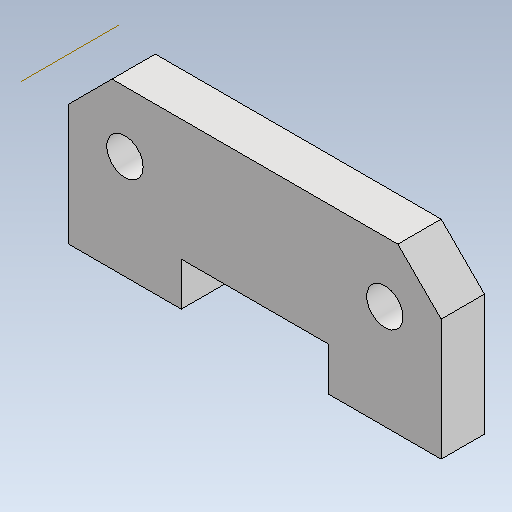
# Autodesk Inventor part: bed-hinge
Saved by Autodesk Inventor 2025 (Build 290162000, 162)
## iProperties
Created: 2025-08-20
Part Number: bed-hinge
Material: Generic
Document SubType Name: Modeling
Designer: HP
Density: 1 g/cm^3
Appearance: Default
Author: HP
Autodesk Inventor part; units mm, degrees
ref_plane "YZ Plane" through (0, 0, 0) normal (1, 0, 0) x (0, 1, 0)
ref_plane "XZ Plane" through (0, 0, 0) normal (0, 1, 0) x (-1, 0, 0)
ref_plane "XY Plane" through (0, 0, 0) normal (0, 0, 1) x (1, 0, 0)
sketch "Sketch1" plane through (0, 0, 0) normal (0, 0, 1) x (1, 0, 0)
  line L0 (6.5, 0) -> (-36.5, 0)
  line L1 (0, 14) -> (0, 0) construction
  circle A0 centre (0, 7) radius 2.1
  line L2 (-6.5, -5) -> (6.5, -5)
  line L3 (6.5, -5) -> (6.5, 14)
  line L4 (6.5, 0) -> (-6.5, 0)
  line L5 (-6.5, 0) -> (-6.5, -5)
  line L6 (-6.5, -5) -> (6.5, 0) construction
  line L7 (6.5, -5) -> (-6.5, 0) construction
  circle A1 centre (-30, 7) radius 2.1
  line L8 (-30, 14) -> (-30, 0) construction
  line L9 (6.5, 14) -> (-36.5, 14)
  line L10 (-36.5, -5) -> (-23.5, -5)
  line L11 (-23.5, -5) -> (-23.5, 0)
  line L12 (-23.5, 0) -> (-36.5, 0)
  line L13 (-36.5, 14) -> (-36.5, -5)
  line L14 (-36.5, -5) -> (-23.5, 0) construction
  line L15 (-23.5, -5) -> (-36.5, 0) construction
  line L16 (-15, 14) -> (-15, 0) construction
  point P0 (0, -2.5)
  point P1 (-6.5, 0)
  point P2 (-30, -2.5)
  point P3 (-23.5, 0)
  point P4 (-36.5, 0)
  point P5 (-30, 7)
  point P6 (-23.5, 0)
  point P7 (-6.5, 0)
  dimension "d1" = 4.2
  dimension "d4" = 7
  dimension "d5" = 5
  dimension "d6" = 13
  dimension "d8" = 4.2
  dimension "d11" = 5
  dimension "d12" = 13
  dimension "d15" = 30
  constraints: 34 end point, 9 midpoint, 6 point on line, 4 parallel, 4 perpendicular, 3 horizontal, 2 centre point, 2 vertical, 1 collinear, 1 horizontal alignment, 1 symmetric about line, 1 vertical alignment, 1 other
  measures "d1" diameter of A0
  measures "d4" distance from line of L0 A0.centre
  measures "d5" distance between parallel lines of L0 L2
  measures "d6" distance between parallel lines of L3 L5
  measures "d8" diameter of A1
  measures "d11" distance between parallel lines of L12 L10
  measures "d12" distance between parallel lines of L11 L13
  measures "d15" distance of A0.centre point (-30, 7)
extrude "Extrusion1" add sketch "Sketch1" along normal blind 5
chamfer "Chamfer1" distance 5 angle 45 2 edges at (6.5, 14, 2.5) (-36.5, 14, 2.5)
equation "\"d8\" = d1"
equation "\"d11\" = d5"
equation "\"d12\" = d6"
body "Solid1"
